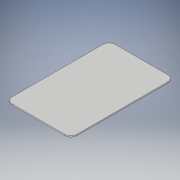
# Autodesk Inventor part: Plastic card
Saved by Autodesk Inventor 2018 (Build 220112000, 112)
## iProperties
Created: 2019-10-16
Part Number: Plastic card
Material: Generic
Document SubType Name: Modeling
Designer: Jacob
Density: 1 g/cm^3
Appearance: Default
Author: Jacob
Autodesk Inventor part; units mm, degrees
ref_plane "YZ Plane" through (0, 0, 0) normal (1, 0, 0) x (0, 1, 0)
ref_plane "XZ Plane" through (0, 0, 0) normal (0, 1, 0) x (-1, 0, 0)
ref_plane "XY Plane" through (0, 0, 0) normal (0, 0, 1) x (1, 0, 0)
sketch "Sketch1" plane through (0, 0, 0) normal (0, 1, 0) x (-1, 0, 0)
  line L0 (26.9875, 42.8625) -> (-26.9875, 42.8625)
  line L1 (-26.9875, 42.8625) -> (-26.9875, -42.8625)
  line L2 (-26.9875, -42.8625) -> (26.9875, -42.8625)
  line L3 (26.9875, -42.8625) -> (26.9875, 42.8625)
  line L4 (26.9875, 42.8625) -> (-26.9875, -42.8625) construction
  line L5 (-26.9875, 42.8625) -> (26.9875, -42.8625) construction
  point P0 (0, 0)
  dimension "d0" = 85.725
  dimension "d1" = 53.975
  constraints: 12 end point, 2 midpoint, 2 parallel, 1 horizontal, 1 perpendicular
  measures "d0" distance of L2.end L0.start
  measures "d1" distance of L1.end L2.end
extrude "Extrusion1" add sketch "Sketch1" along normal blind 1
fillet "Fillet1" radius 5 4 edges at (26.9875, 0.5, 42.8625) (-26.9875, 0.5, 42.8625) (-26.9875, 0.5, -42.8625) (26.9875, 0.5, -42.8625)
body "Solid1"
